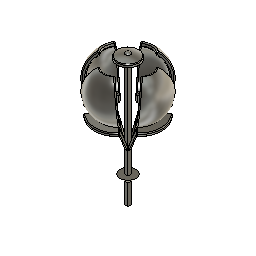
Pawn upper part (Autodesk Fusion 360 design; units mm, degrees)
Autodesk Fusion 360 part; units mm, degrees
note: some values were not read from the file. Chosen so that the rebuilt part matches the saved one: which bodies a step acts on; which face or edge a step refers to.
sphere "SpherePrimitive1" add diameter 30 placed x (1, 0, 0) y (0, 1, 0) z (0, 0, 1) at (0, 0, 0) makes body 1
shell "Shell1" thickness 2 removed faces 0 bodies 1
sketch "Sketch2" plane through (0, 0, 0) normal (0, 1, 0) x (1, 0, 0)
  line L0 (-15, 15) -> (16, 15)
  line L1 (16, 15) -> (16, 12.7)
  line L2 (16, 12.7) -> (-15, 12.7)
  line L3 (-15, 12.7) -> (-15, 15)
  dimension "d3" = 2.3
  constraint horizontal L0
  constraint vertical L1
  constraint horizontal L2
  constraint vertical L3
  measures "d3" distance of L0.start L2.end
extrude "Extrude1" cut sketch "Sketch2" along normal mid plane 80 bodies 1
sketch "Sketch3" plane through (0, 0, 0) normal (0, 0, 1) x (1, 0, 0)
  circle A0 centre (0, 0) radius 6.5
  circle A1 centre (0, 0) radius 6.25
  dimension "d6" = 13
  dimension "d7" = 12.5
  constraint coincident A0.centre A1.centre
  measures "d6" diameter of A0
  measures "d7" diameter of A1
extrude "Extrude2" cut sketch "Sketch3" along normal blind 30 bodies 1 makes body 2 at (7.4978, -12.9866, 0.3622)
move_body "Move1" bodies 1 to x (1, 0, 0) y (0, 1, 0) z (0, 0, 1) at (72, 0, 0)
sketch "Sketch4" plane through (0, 0, 0) normal (0, 1, 0) x (1, 0, 0)
  line L0 (0, 15) -> (0.25, 15)
  line L1 (0.25, 15) -> (0.25, -35)
  line L2 (0.25, -35) -> (0, -35)
  line L3 (0, 15) -> (-0.25, 15)
  line L4 (-0.25, 15) -> (-0.25, -35)
  line L5 (-0.25, -35) -> (0, -35)
  line L6 (0, -35) -> (0, 15)
  dimension "d10" = 0.25
  dimension "d11" = 50
  dimension "d12" = 50
  constraint horizontal L0
  constraint vertical L1
  constraint horizontal L2
  constraint horizontal L3
  constraint vertical L4
  constraint horizontal L5
  constraint vertical L6
  measures "d10" distance of L0.start L0.end
  measures "d11" distance of L0.start L2.end
  measures "d12" distance of L0.start L2.end
extrude "Extrude3" cut sketch "Sketch4" along normal mid plane 600 bodies 2 makes body 3 at (-8.9351, -12.043, 0.3622)
sketch "Sketch5" plane through (0, 0, 0) normal (1, 0, 0) x (0, 1, 0)
  line L0 (0, -15) -> (-0.25, -15)
  line L1 (-0.25, -15) -> (-0.25, 20)
  line L2 (-0.25, 20) -> (0, 20)
  line L3 (0, 20) -> (0, -15)
  line L4 (0, -15) -> (0.25, -15)
  line L5 (0.25, -15) -> (0.25, 20)
  line L6 (0.25, 20) -> (0, 20)
  line L7 (0, 20) -> (0, -15)
  dimension "d15" = 0.25
  dimension "d16" = 35
  dimension "d17" = 35
  constraint horizontal L0
  constraint vertical L1
  constraint horizontal L2
  constraint vertical L3
  constraint horizontal L4
  constraint vertical L5
  constraint horizontal L6
  constraint vertical L7
  measures "d15" distance of L0.start L0.end
  measures "d16" distance of L0.start L2.end
  measures "d17" distance of L0.start L2.end
extrude "Extrude4" cut sketch "Sketch5" along normal mid plane 40 bodies 2 3 makes body 5 at (-3.1091, 14.6698, 0.3622) makes body 4 at (13.8058, 5.8538, 0.3622)
sketch "Sketch6" plane through (0, 0, 0) normal (0, 0, 1) x (1, 0, 0)
  line L0 (110, 5) -> (112, 5)
  line L1 (112, 5) -> (112, 3)
  line L2 (112, 3) -> (110, 3)
  line L3 (110, 3) -> (110, 5)
  constraint horizontal L0
  constraint vertical L1
  constraint horizontal L2
  constraint vertical L3
extrude "Extrude5" add sketch "Sketch6" along normal blind 70.7 separate body makes body 6
move_body "Move2" bodies 1 to x (1, 0, 0) y (0, 1, 0) z (0, 0, 1) at (39, 0, 64)
move_body "Align1" bodies 1 to x (1, 0, 0) y (0, 1, 0) z (0, 0, 1) at (0, 4, -4.699)
sketch "Sketch7" plane through (0, 0, 0) normal (0, 1, 0) x (1, 0, 0)
  line L0 (135, -15) -> (131.5, -15)
  line L1 (135, -15) -> (135, -11.5)
  line L2 (131.5, -15) -> (135, -11.5)
  dimension "d22" = 3.5
  dimension "d23" = 3.5
  constraint horizontal L0
  constraint perpendicular L0 L1
  measures "d22" distance of L0.start L0.end
  measures "d23" distance of L0.start L1.end
sketch "Sketch8" plane through (0, 0, 0) normal (0, 1, 0) x (1, 0, 0)
  line L0 (135, -15) -> (136, -15)
  line L1 (136, -15) -> (136, -12.5053)
  line L2 (136, -12.5053) -> (135, -12.5053)
  line L3 (135, -12.5053) -> (135, -15)
  dimension "d24" = 1
  constraint horizontal L0
  constraint vertical L1
  constraint horizontal L2
  constraint vertical L3
  measures "d24" distance of L0.start L0.end
revolve "Revolve1" add sketch "Sketch8" sketch "Sketch7" angle 360 about axis through (136, 0, 15) along (0, 0, -1) separate body of sketch 2 makes body 7
move_body "Move3" bodies 7 to x (1, 0, 0) y (0, 1, 0) z (0, 0, 1) at (-25, 4, 0)
sphere "SpherePrimitive2" add diameter 4 placed x (1, 0, 0) y (0, 0, -1) z (0, 1, 0) at (135, 0, 10) separate body makes body 8
move_body "Move4" bodies 8 to x (1, 0, 0) y (0, 1, 0) z (0, 0, 1) at (-24, 4, 63)
combine "Combine1" operation add target body 1 tool bodies 8 6 7 makes body 9 at (112, 4.0001, 52.1333)
sketch "Sketch10" plane through (0, 0, 0) normal (0, 0, 1) x (1, 0, 0)
  line L0 (130, 0) -> (131, 0)
  line L1 (131, 0) -> (131, 1)
  line L2 (131, 1) -> (130, 1)
  line L3 (130, 1) -> (130, 0)
  constraint horizontal L0
  constraint vertical L1
  constraint horizontal L2
  constraint vertical L3
extrude "Extrude6" add sketch "Sketch10" along normal blind 18 separate body makes body 10
move_body "Move5" bodies 10 to x (1, 0, 0) y (0, 1, 0) z (0, 0, 1) at (0, 0, 27)
move_body "Move6" bodies 10 to x (0.913545, 0, -0.406737) y (0, 1, 0) z (0.406737, 0, 0.913545) at (0.3437, 0, 55.6168)
move_body "Move7" bodies 2 to x (1, 0, 0) y (0, 1, 0) z (0, 0, 1) at (33.4631, 0, 39.9441)
move_body "Move8" bodies 2 to x (0.707107, 0.707107, 0) y (-0.707107, 0.707107, 0) z (0, 0, 1) at (9.8011, -23.662, 0)
move_body "Move9" bodies 2 to x (1, 0, 0) y (0, 1, 0) z (0, 0, 1) at (0, 0.5, 0)
move_body "Move10" bodies 2 to x (0.993572, 0, -0.113203) y (0, 1, 0) z (0.113203, 0, 0.993572) at (-2.2144, 0, 15.0032)
move_body "Move11" bodies 2 to x (1, 0, 0) y (0, 1, 0) z (0, 0, 1) at (85, 0, 10)
move_body "Move12" bodies 10 to x (1, 0, 0) y (0, 1, 0) z (0, 0, 1) at (-13, 0, 0)
move_body "Move13" bodies 2 to x (1, 0, 0) y (0, 1, 0) z (0, 0, 1) at (3, 0, 0)
move_body "Move14" bodies 2 to x (1, 0, 0) y (0, 1, 0) z (0, 0, 1) at (-1, 0, -5)
combine "Combine2" operation add target body 2 tool bodies 10
move_body "Move15" bodies 2 to x (1, 0, 0) y (0, 1, 0) z (0, 0, 1) at (12, 3.5, 3)
combine "Combine3" operation add target body 1 tool bodies 9 makes body 11 at (112, 4.0001, 52.1333)
mirror "Mirror1" about plane through (110, 3, 0) normal (-1, 0, 0) of bodies 2 makes body 12
mirror "Mirror2" about plane through (110, 3, 42.85) normal (-0.707107, 0.707107, 0) of bodies 12 makes body 13
mirror "Mirror3" about plane through (110, 5, 0) normal (0, 1, 0) of bodies 13 makes body 14
move_body "Move16" bodies 2 to x (1, 0, 0) y (0, 1, 0) z (0, 0, 1) at (-18, 0, 0)
move_body "Move17" bodies 12 to x (1, 0, 0) y (0, 1, 0) z (0, 0, 1) at (20, 0, 0)
move_body "Move18" bodies 13 to x (1, 0, 0) y (0, 1, 0) z (0, 0, 1) at (0, 20, 0)
move_body "Move19" bodies 14 to x (1, 0, 0) y (0, 1, 0) z (0, 0, 1) at (0, -22, 0)
delete_body "RemoveBody1" bodies 3
delete_body "RemoveBody2" bodies 5
delete_body "RemoveBody3" bodies 4
move_body "Move20" bodies 1 to x (1, 0, 0) y (0, 1, 0) z (0, 0, 1) at (0, 0, -1)
move_body "Move21" bodies 13 to x (1, 0, 0) y (0, 1, 0) z (0, 0, 1) at (0, 0, -1)
move_body "Move22" bodies 14 to x (1, 0, 0) y (0, 1, 0) z (0, 0, 1) at (0, 0, -1)
move_body "Move23" bodies 12 to x (1, 0, 0) y (0, 1, 0) z (0, 0, 1) at (0, 0, -1)
move_body "Move24" bodies 2 to x (1, 0, 0) y (0, 1, 0) z (0, 0, 1) at (0, 0, -1)
combine "Combine4" operation add target body 1 tool bodies 12 14 2 13 11
split "Split1" by plane through (112, 5, 0) normal (1, 0, 0) bodies 1 makes body 15 at (114.5969, -16.0607, 56.6143) makes body 16 at (117.0835, 23.2145, 56.7107) makes body 17 at (129.0872, 12.1746, 56.8391) makes body 18 at (114.7222, 4, 14.2222) makes body 19 at (115.9815, 4.9825, 70.2684)
split "Split2" by plane through (126.3587, 15.3137, 44.0033) normal (-0.113203, 0, -0.993572) bodies 17 makes body 20 at (116.7004, 3.8333, 39.5573)
move_body "Move25" bodies 20 to x (1, 0, 0) y (0, 1, 0) z (0, 0, 1) at (50, 0, 0)
split "Split3" by plane through (112, 3, 0) normal (0, -1, 0) bodies 15 1 makes body 21 at (105.168, -15.3227, 56.6984) makes body 22 at (111.0659, -0.9796, 72.4502) makes body 23 at (107.9998, 1.7968, 14.2222) makes body 24 at (90.9393, 0.4031, 56.6143)
split "Split4" by plane through (110, 3, 0) normal (-1, 0, 0) bodies 24 1 makes body 25 at (92.9745, 12.2692, 56.8462) makes body 26 at (106.0204, 3.9341, 72.4502) makes body 27 at (108.768, 6.9787, 14.2222) makes body 28 at (102.6168, 21.95, 56.8548)
split "Split5" by plane through (110, 5, 0) normal (0, 1, 0) bodies 28 1 16 makes body 29 at (111, 22.484, 65.5083) makes body 30 at (111.4166, 7.6988, 14.2222) makes body 31 at (112, 9.1441, 71.6244)
delete_body "RemoveBody4" bodies 15
delete_body "RemoveBody5" bodies 16
delete_body "RemoveBody6" bodies 20
delete_body "RemoveBody7" bodies 21
delete_body "RemoveBody8" bodies 24
delete_body "RemoveBody9" bodies 25
delete_body "RemoveBody10" bodies 28
delete_body "RemoveBody11" bodies 29
combine "Combine5" operation add target body 26 tool bodies 31 19 22 1 23 27 30 18
sketch "Sketch11" plane through (112, 0, 0) normal (1, 0, 0) x (0, 1, 0)
  spline S0 degree 2 poles (5, 11.9142) (4.4142, 11.5) (4, 11.5) knots 0.342577 0.342577 0.342577 0.565698 0.565698 0.565698 weights 1.314479 1.259649 1
  spline S1 degree 2 poles (4, 11.5) (3.5858, 11.5) (3, 11.9142) knots 0.565698 0.565698 0.565698 0.788818 0.788818 0.788818 weights 1 1.259649 1.314479
  line L0 (3, 11.9142) -> (3, 0)
  line L1 (3, 0) -> (5, 0)
  line L2 (5, 0) -> (5, 11.9142)
  line L3 (12.5, 0) -> (13.5, 0)
  line L4 (13.5, 0) -> (13.5, 21)
  line L5 (13.5, 21) -> (12.5, 21)
  line L6 (12.5, 21) -> (12.5, 0)
  dimension "d81" = 1
  dimension "d82" = 21
  constraint horizontal L3
  constraint vertical L4
  constraint horizontal L5
  constraint vertical L6
  measures "d81" distance of L3.start L3.end
  measures "d82" distance of L3.start L5.end
extrude "Extrude7" add sketch "Sketch11" along normal blind 1 separate body contours L3 L4 L5 L6 makes body 32
move_body "Move26" bodies 32 to x (1, 0, 0) y (0, 1, 0) z (0, 0, 1) at (0, 0, 17)
split "Split6" by plane through (111, 4, 15) normal (0, 0, 1) bodies 26 makes body 33 at (115.8959, 5.0152, 72.4431)
move_body "Move27" bodies 33 to x (1, 0, 0) y (0, 1, 0) z (0, 0, 1) at (0, 0, 2)
sketch "Sketch12" plane through (0, 0, 17) normal (0, 0, -1) x (1, 0, 0)
  line L0 (112, -5) -> (112, -3)
  line L1 (112, -3) -> (110, -3)
  line L2 (110, -3) -> (110, -5)
  line L3 (110, -5) -> (112, -5)
  line L4 (112, -5) -> (110, -5)
  line L5 (110, -5) -> (110, -3)
  line L6 (110, -3) -> (112, -3)
  line L7 (112, -3) -> (112, -5)
  constraint horizontal L4
  constraint vertical L5
  constraint horizontal L6
  constraint vertical L7
  constraint coincident L1.end L2.start
  constraint coincident L0.start L3.end
extrude "Extrude8" add sketch "Sketch12" along normal blind 1 bodies 33
move_body "Move28" bodies 33 to x (1, 0, 0) y (0, 1, 0) z (0, 0, 1) at (0, 0, -1)
move_body "Move29" bodies 32 to x (0.927184, 0, -0.374607) y (0, 1, 0) z (0.374607, 0, 0.927184) at (1.8599, 0, 43.5684)
move_body "Move30" bodies 32 to x (1, 0, 0) y (0, 1, 0) z (0, 0, 1) at (-1, 0, 9)
move_body "Move31" bodies 32 to x (1, 0, 0) y (0, 1, 0) z (0, 0, 1) at (0, -9, 0)
combine "Combine6" operation add target body 33 tool bodies 26
combine "Combine7" operation add target body 17 tool bodies 32
move_body "Move32" bodies 17 to x (1, 0, 0) y (0, 1, 0) z (0, 0, 1) at (0, 0, 1)
mirror "Mirror4" about plane through (112, 3, 43.2929) normal (0.707107, 0.707107, 0) of bodies 17 merged
mirror "Mirror5" about plane through (110, 3, 43.2929) normal (-0.707107, 0.707107, 0) of bodies 17 merged
split "Split7" by plane through (110, 5, 1) normal (0, 1, 0) bodies 17 makes body 34 at (93.05, 12.3832, 57.8548) makes body 35 at (128.95, 12.3832, 57.8548) makes body 36 at (116.6229, 23.4085, 57.6886)
delete_body "RemoveBody12" bodies 17
delete_body "RemoveBody13" bodies 34
delete_body "RemoveBody14" bodies 35
sketch "Sketch13" plane through (0, 0, 0) normal (0, 0, 1) x (1, 0, 0)
  circle A0 centre (0, 0) radius 15
  dimension "d112" = 30
  constraint coincident A0.centre origin
  measures "d112" diameter of A0
extrude "Extrude9" add sketch "Sketch13" along normal blind 2 separate body makes body 37
sketch "Sketch14" plane through (0, 0, 2) normal (0, 0, 1) x (-1, 0, 0)
  circle A0 centre (0, 0) radius 15
  circle A1 centre (0, 0) radius 6.5
  dimension "d115" = 13
  constraint coincident A0.centre A1.centre
  measures "d115" diameter of A1
extrude "Extrude10" cut sketch "Sketch14" against normal blind 4 contours A1 bodies 37
sketch "Sketch15" plane through (0, 0, 2) normal (0, 0, 1) x (-1, 0, 0)
  circle A0 centre (0, 0) radius 6.5
  circle A1 centre (0, 0) radius 15
  line L0 (0.5, 6) -> (-0.5, 6)
  line L1 (-0.5, 6) -> (-0.5, 15.6766)
  line L2 (-0.5, 15.6766) -> (0.5, 15.6766)
  line L3 (0.5, 15.6766) -> (0.5, 6)
  line L4 (-5.5, -0.5) -> (-25.5, -0.5)
  line L5 (-25.5, -0.5) -> (-25.5, 0.5)
  line L6 (-25.5, 0.5) -> (-5.5, 0.5)
  line L7 (-5.5, 0.5) -> (-5.5, -0.5)
  dimension "d118" = 1
  dimension "d119" = 20
  dimension "d120" = 1
  constraint horizontal L0
  constraint vertical L1
  constraint horizontal L2
  constraint vertical L3
  constraint horizontal L4
  constraint vertical L5
  constraint horizontal L6
  constraint vertical L7
  measures "d118" distance of L0.start L0.end
  measures "d119" distance of L4.start L4.end
  measures "d120" distance of L4.start L6.end
extrude "Extrude11" cut sketch "Sketch15" against normal blind 4 contours A0 L0 L1 L3 | A0 A1 L1 L3 | A0 A1 L4 L6 | A0 L4 L6 L7 | A1 L1 L2 L3 | A1 L4 L5 L6 bodies 37 makes body 38 at (8.5866, -8.5866, 2)
delete_body "RemoveBody15" bodies 37
move_body "Move33" bodies 38 to x (1, 0, 0) y (0, 1, 0) z (0, 0, 1) at (70, 0, 0)
move_body "Move34" bodies 38 to x (-0.707107, 0.707107, 0) y (-0.707107, -0.707107, 0) z (0, 0, 1) at (119.4975, -49.4975, 0)
move_body "Move35" bodies 38 to x (1, 0, 0) y (0, 0.993572, -0.113203) z (0, 0.113203, 0.993572) at (0, 0.0321, 0.566)
move_body "Move36" bodies 38 to x (1, 0, 0) y (0, 1, 0) z (0, 0, 1) at (41, 9, 45.8)
move_body "Move37" bodies 38 to x (1, 0, 0) y (0, 1, 0) z (0, 0, 1) at (0, -1, 0.3)
fillet "Fillet1" radius 0.5 6 edges at (105.173, 1.7399, 72.9369) (105.173, 6.2601, 70.7) (111, 17.5439, 71.5982) (111, 17.2881, 69.3525) (111, 23.1621, 46.9551) (111, 22.9357, 44.968) on bodies 33 36 38
fillet "Fillet2" radius 0.5 20 edges at (102.1112, 18.4963, 55.7323) (106.5386, 15.6185, 69.584) (106.584, 15.6664, 70.4054) (106.4091, 15.9543, 71.3875) (100.576, 20.3123, 58.1095) (121.424, 20.3123, 58.1095) (115.5909, 15.9543, 71.3875) (115.416, 15.6664, 70.4054) (115.4614, 15.6185, 69.584) (119.8888, 18.4963, 55.7323) (103.9388, 15.7505, 45.7866) (100.8565, 18.8296, 45.5832) (100.7528, 19.0292, 46.4195) (100.8565, 19.0228, 47.2794) (103.9388, 15.9769, 47.7738) (118.0612, 15.9769, 47.7738) (121.1435, 19.0228, 47.2794) (121.2472, 19.0292, 46.4195) (121.1435, 18.8296, 45.5832) (118.0612, 15.7505, 45.7866) on bodies 36 38
combine "Combine8" operation add target body 36 tool bodies 38
mirror "Mirror6" about plane through (110, 5, 43.2929) normal (0.707107, 0.707107, 0) of bodies 36 makes body 39
mirror "Mirror7" about plane through (110, 3, 43.2929) normal (-0.707107, 0.707107, 0) of bodies 39 makes body 40
mirror "Mirror8" about plane through (110, 5, 43.2929) normal (0.707107, 0.707107, 0) of bodies 40 makes body 41
combine "Combine9" operation add target body 33 tool bodies 36 41 39 40
equation "d126 = -45 deg - 90.0 deg"
